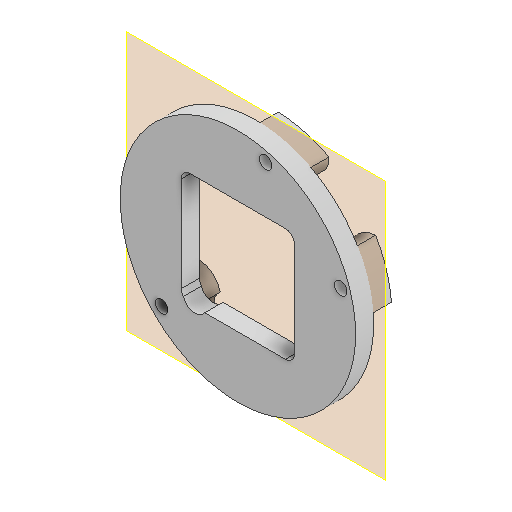
# Autodesk Inventor part: Anglerfish_flipped_LidMoun
Saved by Autodesk Inventor 2022 (Build 260153000, 153)
## iProperties
Created: 2022-04-02
Part Number: Anglerfish_flipped_LidMoun
Material: Generic
Document SubType Name: Modeling
Designer: Prakash Lab
Density: 1 g/cm^3
Appearance: Default
Author: Prakash Lab
Autodesk Inventor part; units mm, degrees
ref_plane "YZ Plane" through (0, 0, 0) normal (1, 0, 0) x (0, 1, 0)
ref_plane "XZ Plane" through (0, 0, 0) normal (0, 1, 0) x (-1, 0, 0)
ref_plane "XY Plane" through (0, 0, 0) normal (0, 0, 1) x (1, 0, 0)
ref_plane "Work Plane1" through (0, 0, 0) normal (0, 0, 1) x (1, 0, 0)
sketch "Sketch1" plane through (0, 0, 0) normal (0, 0, 1) x (1, 0, 0)
  circle A0 centre (0, 0) radius 25.9979 projected
  circle A1 centre (-9.4998, -11.0022) radius 2.6601 projected
  circle A2 centre (0.0001, -0.0022) radius 3.8801 projected
  circle A3 centre (0.0001, -0.0022) radius 6.7754 projected
  line L0 (10.5001, -12.5022) -> (-10.4999, -12.5022)
  line L1 (-12.4999, -10.5022) -> (-12.4999, 10.4978)
  line L2 (-10.4999, 12.4978) -> (10.5001, 12.4978)
  line L3 (12.5001, 10.4978) -> (12.5001, -10.5022)
  line L4 (12.5001, -12.5022) -> (-12.4999, 12.4978) construction
  line L5 (-12.4999, -12.5022) -> (12.5001, 12.4978) construction
  arc A4 (-10.4999, 12.4978) -> (-12.4999, 10.4978) centre (-10.4999, 10.4978) ccw
  arc A5 (-12.4999, -10.5022) -> (-10.4999, -12.5022) centre (-10.4999, -10.5022) ccw
  arc A6 (10.5001, -12.5022) -> (12.5001, -10.5022) centre (10.5001, -10.5022) ccw
  arc A7 (12.5001, 10.4978) -> (10.5001, 12.4978) centre (10.5001, 10.4978) ccw
  point P0 (0, 0)
  point P1 (-7.3029, -12.5022)
  point P2 (-12.0467, -11.77)
  dimension "d17" = 25
  dimension "d18" = 25
  dimension "d19" = 2
  constraints: 12 end point, 8 point on circle, 8 point on line, 8 tangent, 4 centre point, 3 equal radius, 2 midpoint, 2 parallel, 1 horizontal, 1 perpendicular
  measures "d17" distance of L4.end L5.end
  measures "d18" distance of L5.start L4.end
  measures "d19" radius of A4
extrude "Extrusion1" add sketch "Sketch1" along normal blind 4 contours A0
sketch "Skizze4" plane through (0, 0, 4) normal (0, 0, 1) x (1, 0, 0)
  spline S0 degree 2 poles (24.1427, 2.2394) (24.731, 1.8489) (25.3785, 0.5587) (25.3785, -0.3311) knots 0 0 0 1 2 2 2 construction
  spline S1 degree 2 poles (25.3785, -0.3311) (25.3785, -1.1665) (24.7013, -2.5111) (24.1328, -2.8867) knots 0 0 0 1 2 2 2 construction
  spline S2 degree 2 poles (24.1328, -2.8867) (23.6682, -3.1784) (22.7141, -3.3761) (21.9726, -3.3761) knots 0 0 0 1 2 2 2 construction
  line L0 (21.9726, -3.3761) -> (20.5687, -3.3761) construction
  line L1 (20.5687, -3.3761) -> (20.5687, 2.7239) construction
  line L2 (20.5687, 2.7239) -> (21.9578, 2.7239) construction
  spline S3 degree 2 poles (21.9578, 2.7239) (22.8179, 2.7239) (23.7967, 2.4668) (24.1427, 2.2394) knots 0 0 0 1 2 2 2 construction
  spline S4 degree 2 poles (19.1896, -2.9312) (18.8979, -3.1982) (18.1564, -3.4849) (17.5978, -3.4849) knots 0 0 0 1 2 2 2 construction
  spline S5 degree 2 poles (17.5978, -3.4849) (16.9354, -3.4849) (16.0061, -3.2081) (15.5958, -3.0103) knots 0 0 0 1 2 2 2 construction
  line L3 (15.5958, -3.0103) -> (15.5958, -1.992) construction
  line L4 (15.5958, -1.992) -> (15.6551, -1.992) construction
  spline S6 degree 2 poles (15.6551, -1.992) (16.0555, -2.3677) (17.0689, -2.7829) (17.5385, -2.7829) knots 0 0 0 1 2 2 2 construction
  spline S7 degree 2 poles (17.5385, -2.7829) (18.2108, -2.7829) (18.8979, -2.2243) (18.8979, -1.7646) knots 0 0 0 1 2 2 2 construction
  spline S8 degree 2 poles (18.8979, -1.7646) (18.8979, -1.3988) (18.5371, -0.944) (18.1465, -0.8303) knots 0 0 0 1 2 2 2 construction
  spline S9 degree 2 poles (18.1465, -0.8303) (17.8648, -0.7513) (17.3952, -0.6425) (17.0442, -0.5535) knots 0 0 0 1 2 2 2 construction
  spline S10 degree 2 poles (17.0442, -0.5535) (16.7278, -0.4695) (16.2285, -0.2174) (16.0358, -0.0147) knots 0 0 0 1 2 2 2 construction
  spline S11 degree 2 poles (16.0358, -0.0147) (15.8479, 0.188) (15.6403, 0.7317) (15.6403, 1.0876) knots 0 0 0 1 2 2 2 construction
  spline S12 degree 2 poles (15.6403, 1.0876) (15.6403, 1.8291) (16.797, 2.8326) (17.6918, 2.8326) knots 0 0 0 1 2 2 2 construction
  spline S13 degree 2 poles (17.6918, 2.8326) (18.2059, 2.8326) (19.1154, 2.6299) (19.5059, 2.4372) knots 0 0 0 1 2 2 2 construction
  line L5 (19.5059, 2.4372) -> (19.5059, 1.4683) construction
  line L6 (19.5059, 1.4683) -> (19.4466, 1.4683) construction
  spline S14 degree 2 poles (19.4466, 1.4683) (19.155, 1.7352) (18.2454, 2.1307) (17.7461, 2.1307) knots 0 0 0 1 2 2 2 construction
  spline S15 degree 2 poles (17.7461, 2.1307) (17.1826, 2.1307) (16.4856, 1.6017) (16.4856, 1.1717) knots 0 0 0 1 2 2 2 construction
  spline S16 degree 2 poles (16.4856, 1.1717) (16.4856, 0.7861) (16.8959, 0.3264) (17.2815, 0.2226) knots 0 0 0 1 2 2 2 construction
  spline S17 degree 2 poles (17.2815, 0.2226) (17.5385, 0.1534) (18.285, -0.0246) (18.5321, -0.0987) knots 0 0 0 1 2 2 2 construction
  spline S18 degree 2 poles (18.5321, -0.0987) (19.1599, -0.2915) (19.7432, -1.0676) (19.7432, -1.6361) knots 0 0 0 1 2 2 2 construction
  spline S19 degree 2 poles (19.7432, -1.6361) (19.7432, -1.997) (19.4516, -2.689) (19.1896, -2.9312) knots 0 0 0 1 2 2 2 construction
  circle A0 centre (-9.9998, 17.4978) radius 1.3999 construction
  circle A1 centre (10.0001, 17.4979) radius 1.4 construction
  circle A2 centre (10.0001, -17.5021) radius 1.4 construction
  circle A3 centre (-9.9998, -17.5021) radius 1.4001 construction
  arc A4 (-25.1198, 6.6998) -> (-24.1417, 5.4917) centre (-24.1417, 6.4917) ccw construction
  line L7 (-24.1417, 5.4917) -> (-17.7002, 5.4917) construction
  arc A5 (-15.7002, 3.4917) -> (-17.7002, 5.4917) centre (-17.7002, 3.4917) ccw construction
  line L8 (-15.7002, 3.4917) -> (-15.7002, -4.496) construction
  arc A6 (-17.7002, -6.496) -> (-15.7002, -4.496) centre (-17.7002, -4.496) ccw construction
  line L9 (-17.7002, -6.496) -> (-23.8502, -6.496) construction
  arc A7 (-23.8502, -6.496) -> (-24.8235, -7.7254) centre (-23.8502, -7.496) ccw construction
  arc A8 (-24.8235, -7.7254) -> (-25.1198, 6.6998) centre (0, 0) ccw construction
  circle A9 centre (-9.4998, -11.0022) radius 2.6601 construction
  circle A10 centre (-16.8291, -16.0482) radius 1.4 construction
  circle A11 centre (6.1284, 23.0202) radius 1.4 construction
  circle A12 centre (22.7119, 7.1872) radius 1.4 construction
  circle A13 centre (0.0001, -0.0022) radius 6.5 construction
  point P0 (0, 0)
hole "Bohrung1" at (6.1284, 23.0202, 4) at (22.7119, 7.1872, 4) at (-16.8291, -16.0482, 4) direction (0, 0, -1) diameter 2.8 end through all
sketch "Skizze6" plane through (0, 0, 0) normal (0, 0, -1) x (-1, 0, 0)
  circle A0 centre (-22.7119, 7.1872) radius 1.4 projected
  circle A1 centre (-6.1284, 23.0202) radius 1.4 projected
  circle A2 centre (16.8291, -16.0482) radius 1.4 projected
  circle A3 centre (0, 0) radius 25.9979 projected
  line L0 (12.4999, -10.5022) -> (12.4999, 10.4978) projected
  arc A4 (12.0467, -11.77) -> (12.4999, -10.5022) centre (10.4999, -10.5022) ccw projected
  arc A5 (7.3029, -12.5022) -> (12.0467, -11.77) centre (9.4998, -11.0022) ccw projected
  line L1 (-10.5001, -12.5022) -> (7.3029, -12.5022) projected
  arc A6 (-12.5001, -10.5022) -> (-10.5001, -12.5022) centre (-10.5001, -10.5022) ccw projected
  line L2 (-12.5001, 10.4978) -> (-12.5001, -10.5022) projected
  arc A7 (-10.5001, 12.4978) -> (-12.5001, 10.4978) centre (-10.5001, 10.4978) ccw projected
  line L3 (10.4999, 12.4978) -> (-10.5001, 12.4978) projected
  arc A8 (12.4999, 10.4978) -> (10.4999, 12.4978) centre (10.4999, 10.4978) ccw projected
  arc A9 (21.6334, -14.4182) -> (15.4291, -20.9245) centre (16.8291, -16.0482) ccw
  circle A10 centre (-6.1284, 23.0202) radius 1.4 projected
  circle A11 centre (0, 0) radius 25.9979 projected
  arc A12 (-12.1283, 22.9955) -> (-0.9103, 25.982) centre (-6.1284, 23.0202) ccw
  circle A13 centre (-22.7119, 7.1872) radius 1.4 projected
  arc A14 (-25.912, 2.1118) -> (-22.4096, 13.1796) centre (-22.7119, 7.1872) ccw
  point P0 (0, 0)
  point P1 (-25.912, 2.1118)
  point P2 (-0.9103, 25.982)
  dimension "d20" = 6
  dimension "d21" = 6
  constraints: 11 point on circle, 3 centre point, 3 coincident, 2 other
  measures "d20" radius of A12
  measures "d21" radius of A14
extrude "Extrusion4" add sketch "Skizze6" along normal blind 4 contours A12 A3 | A3 A9 | A14 A3
sketch "Skizze7" plane through (0, 0, 0) normal (0, 0, -1) x (-1, 0, 0)
  arc A0 (-25.912, 2.1118) -> (-22.4096, 13.1796) centre (-22.7119, 7.1872) ccw projected
  arc A1 (-25.912, 2.1118) -> (15.4291, -20.9245) centre (0, 0) ccw projected
  arc A2 (21.6334, -14.4182) -> (15.4291, -20.9245) centre (16.8291, -16.0482) ccw projected
  arc A3 (21.6334, -14.4182) -> (-0.9103, 25.982) centre (0, 0) ccw projected
  arc A4 (-12.1283, 22.9955) -> (-0.9103, 25.982) centre (-6.1284, 23.0202) ccw projected
  arc A5 (-12.1283, 22.9955) -> (-22.4096, 13.1796) centre (0, 0) ccw projected
  line L0 (12.4999, -10.5022) -> (12.4999, 10.4978) projected
  arc A6 (12.0467, -11.77) -> (12.4999, -10.5022) centre (10.4999, -10.5022) ccw projected
  arc A7 (7.3029, -12.5022) -> (12.0467, -11.77) centre (9.4998, -11.0022) ccw projected
  line L1 (-10.5001, -12.5022) -> (7.3029, -12.5022) projected
  arc A8 (-12.5001, -10.5022) -> (-10.5001, -12.5022) centre (-10.5001, -10.5022) ccw projected
  line L2 (-12.5001, 10.4978) -> (-12.5001, -10.5022) projected
  arc A9 (-10.5001, 12.4978) -> (-12.5001, 10.4978) centre (-10.5001, 10.4978) ccw projected
  line L3 (10.4999, 12.4978) -> (-10.5001, 12.4978) projected
  arc A10 (12.4999, 10.4978) -> (10.4999, 12.4978) centre (10.4999, 10.4978) ccw projected
  circle A11 centre (8.3387, 18.1787) radius 4
  circle A12 centre (-0.0001, -20) radius 4
  circle A13 centre (-19.3477, -5.0663) radius 4
  circle A14 centre (0, 0) radius 20 construction
  point P0 (0, 0)
  dimension "d24" = 8
  dimension "d25" = 8
  dimension "d26" = 8
  dimension "d29" = 40
  constraints: 4 centre point, 3 point on circle, 1 coincident
  measures "d24" diameter of A11
  measures "d25" diameter of A12
  measures "d26" diameter of A13
  measures "d29" diameter of A14
extrude "Extrusion5" cut sketch "Skizze7" against normal blind 3 contours A11 | A12 | A13
sketch "Skizze8" plane through (0, 0, -4) normal (0, 0, -1) x (-1, 0, 0)
  circle A0 centre (16.8271, -16.0472) radius 2.75 projected
  circle A1 centre (-22.7139, 7.1882) radius 2.75 projected
  circle A2 centre (-6.1303, 23.0212) radius 2.75 projected
  circle A3 centre (-6.1303, 23.0212) radius 3.25
  circle A4 centre (-22.7139, 7.1882) radius 3.25
  circle A5 centre (16.8271, -16.0472) radius 3.25
  circle A6 centre (-10.002, -17.5012) radius 2.75 projected
  circle A7 centre (9.998, -17.5011) radius 2.75 projected
  circle A8 centre (-10.002, 17.4988) radius 2.75 projected
  circle A9 centre (-10.002, 17.4988) radius 3.25
  circle A10 centre (-10.002, -17.5012) radius 3.25
  circle A11 centre (9.998, -17.5011) radius 3.25
  point P0 (0, 0)
  dimension "d30" = 0.5
  dimension "d31" = 0.5
  dimension "d32" = 0.5
  dimension "d33" = 0.5
  dimension "d34" = 0.5
  dimension "d35" = 0.5
  constraints: 6 centre point
  measures "d30" radial gap between concentric circles of A2 A3
  measures "d31" radial gap between concentric circles of A1 A4
  measures "d32" radial gap between concentric circles of A0 A5
  measures "d33" radial gap between concentric circles of A8 A9
  measures "d34" radial gap between concentric circles of A6 A10
  measures "d35" radial gap between concentric circles of A7 A11
extrude "Extrusion6" cut sketch "Skizze8" against normal up to surface (4 mm away) contours A6 | A7 | A8 | A9 | A10 | A11
body "Solid1"
